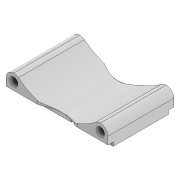
# Autodesk Inventor part: oxybeamBottom
Saved by Autodesk Inventor 2020 (Build 240168000, 168)
## iProperties
Created: 2020-05-15
Part Number: oxybeamBottom
Material: Generic
Document SubType Name: Modeling
Designer: rayan
Density: 1 g/cm^3
Appearance: Default
Author: rayan
Autodesk Inventor part; units mm, degrees
ref_plane "XZ Plane" through (0, 0, 0) normal (0, 1, 0) x (-1, 0, 0)
ref_plane "XY Plane" through (0, 0, 0) normal (0, 0, 1) x (1, 0, 0)
sketch "Sketch1" plane through (0, 0, 0) normal (0, 0, 1) x (1, 0, 0)
  circle A0 centre (0, 0) radius 1.7
  circle A1 centre (0, 0) radius 3
  dimension "d0" = 3.4
  dimension "d1" = 6
  constraints: 2 centre point, 2 coincident
  measures "d0" diameter of A0
  measures "d1" diameter of A1
extrude "Extrusion1" add sketch "Sketch1" along normal mid plane 26
sketch "Sketch2" plane through (0, 0, 13) normal (0, 0, 1) x (1, 0, 0)
  line L0 (0, 0) -> (-3, 0)
  line L1 (-3, 0) -> (-3, -8)
  line L2 (-3, -8) -> (0, -8)
  line L3 (0, -8) -> (0, 0) construction
  line L4 (0, 0) -> (3, 0)
  line L5 (3, 0) -> (3, -5)
  line L6 (3, -5) -> (0, -5)
  line L7 (0, -5) -> (0, 0) construction
  line L8 (0, -5) -> (0, -8)
  circle A0 centre (0, 0) radius 1.7 projected
  point P0 (1.7, 0)
  point P1 (-1.7, 0)
  dimension "d4" = 3
  dimension "d5" = 8
  dimension "d6" = 3
  dimension "d7" = 5
  constraints: 18 end point, 4 parallel, 3 perpendicular, 2 horizontal
  measures "d4" distance of L2.end L1.end
  measures "d5" distance of L1.end L0.end
  measures "d6" distance of L5.end L6.end
  measures "d7" distance of L4.end L5.end
extrude "Extrusion2" add sketch "Sketch2" against normal up to surface (26 mm away) contours A0 L4 L5 L6 L8 L2 L1 L0
sketch "Sketch3" plane through (0, 0, 13) normal (0, 0, 1) x (1, 0, 0)
  line L0 (-3, 0) -> (-3, -8) projected
  line L1 (3, -5) -> (3, 0) projected
  line L2 (-3, -8) -> (3, -8)
  line L3 (3, -8) -> (3, -3)
  line L4 (3, -3) -> (-3, -3)
  line L5 (-3, -3) -> (-3, -8)
  point P0 (0, 0)
  point P1 (-3, -3)
  dimension "d10" = 5
  constraints: 8 end point, 2 parallel, 1 horizontal, 1 perpendicular, 1 point on line
  measures "d10" distance of L3.end L2.end
extrude "Extrusion3" cut sketch "Sketch3" against normal blind 2.05
mirror "Mirror1" about plane through (0, 0, 0) normal (0, 0, 1) of "Extrusion3"
sketch "Sketch4" plane through (0, -8, 10.95) normal (1, 0, 0) x (0, 0, -1)
  line L0 (0, 3) -> (0, 0) projected
  line L1 (0, 0) -> (21.9, 0) projected
  line L2 (0, 0) -> (21.9, 0)
  line L3 (21.9, 0) -> (21.9, 3.5)
  line L4 (21.9, 3.5) -> (0, 3.5)
  line L5 (0, 3.5) -> (0, 0)
  line L6 (0, 3) -> (21.9, 3) construction
  line L7 (21.9, 5) -> (23.95, 5) projected
  point P0 (10.95, 8)
  point P1 (0, 1.5)
  dimension "d16" = 1.5
  constraints: 8 end point, 2 parallel, 1 horizontal, 1 perpendicular
  measures "d16" distance between parallel lines of L7 L4
extrude "Extrusion4" cut sketch "Sketch4" against normal through all both and the other way through all
sketch "Sketch5" plane through (3, 0, 13) normal (1, 0, 0) x (0, 0, -1)
  line L0 (23.95, -4.5) -> (2.05, -4.5) projected
  line L1 (2.05, -4.5) -> (5.05, -4.5)
  line L2 (23.95, -4.5) -> (23.95, -3) projected
  line L3 (23.95, -4.5) -> (20.95, -4.5)
  line L4 (2.05, -3) -> (0, -3) projected
  line L5 (26, -3) -> (23.95, -3) projected
  line L6 (2.05, -3) -> (23.95, -3)
  arc A0 (20.95, -4.5) -> (5.05, -4.5) centre (13, -24.8175) ccw
  point P0 (13, 0)
  dimension "d17" = 3
  dimension "d18" = 3
  constraints: 6 end point, 2 point on circle, 2 point on line, 1 centre point, 1 collinear, 1 tangent
  measures "d17" distance of L0.end L1.end
  measures "d18" distance of L0.start L3.end
extrude "Extrusion5" [suppressed]
fillet "Fillet1" [suppressed]
ref_plane "Work Plane1" through (17.1, 0, 0) normal (1, 0, 0) x (0, 1, 0)
mirror "Mirror2" about plane through (17.1, 0, 0) normal (1, 0, 0) of "Extrusion1", "Extrusion2", "Extrusion3", "Mirror1", "Extrusion4"
sketch "Sketch7" plane through (3, 0, 13) normal (1, 0, 0) x (0, 0, -1)
  line L0 (23.95, -4.5) -> (23.95, -3) projected
  line L1 (23.95, -3) -> (26, -3) projected
  line L2 (26, 0) -> (26, -3) projected
  line L3 (26, 0) -> (0, 0) projected
  line L4 (0, -3) -> (0, 0) projected
  line L5 (0, -3) -> (2.05, -3) projected
  line L6 (2.05, -3) -> (2.05, -4.5) projected
  line L7 (0, 3) -> (0, 0) projected
  line L8 (26, 0) -> (0, 0) projected
  line L9 (0, 0) -> (26, 0)
  line L10 (26, 0) -> (26, -1.5)
  line L11 (26, -1.5) -> (0, -1.5)
  line L12 (0, -1.5) -> (0, 0)
  line L13 (2.05, -4.5) -> (23.95, -4.5) projected
  point P0 (13, 0)
  point P1 (0, -1.5)
  dimension "d25" = 1.5
  constraints: 8 end point, 3 equal length, 1 perpendicular
  measures "d25" distance between parallel lines of L11 L5
extrude "Extrusion7" add sketch "Sketch7" along normal up to surface (28.2 mm away) contours L13 L6 L5 L4 L11 L2 L1 L0
sketch "Sketch8" plane through (3, -1.5, 13) normal (0, 1, 0) x (1, 0, 0)
  line L0 (28.2, 26) -> (28.2, 0) construction
  line L1 (0, 26) -> (28.2, 26) construction
  line L2 (0, 0) -> (0, 26) construction
  line L3 (0, 0) -> (28.2, 0) construction
  line L4 (-6, 0) -> (0, 0) construction
  line L5 (28.2, 26) -> (0, 0) construction
  line L6 (28.2, 26) -> (28.2, 0) projected
  line L7 (0, 7.2315) -> (28.2, 7.2315)
  line L8 (28.2, 7.2315) -> (28.2, 18.7685)
  line L9 (28.2, 18.7685) -> (0, 18.7685)
  line L10 (0, 18.7685) -> (0, 7.2315)
  line L11 (0, 7.2315) -> (28.2, 18.7685) construction
  line L12 (28.2, 7.2315) -> (0, 18.7685) construction
  point P0 (-3, 13)
  point P1 (14.1, 13)
  dimension "d28" = 11.537
  constraints: 14 end point, 3 midpoint, 2 parallel, 1 horizontal, 1 perpendicular, 1 point on line
  measures "d28" distance of L8.end L7.end
extrude "Extrusion8" [suppressed]
fillet "Fillet2" radius 1.5 2 edges at (31.2, -1.5, 0) (3, -1.5, 0)
fillet "Fillet3" [suppressed]
sketch "Sketch9" plane through (0, 0, -13) normal (0, 0, -1) x (-1, 0, 0)
  arc A0 (3, 0) -> (-3, 0) centre (0, 0) ccw construction
  line L0 (0, 0) -> (0, 3)
  line L1 (0, 3) -> (-1.1, 3)
  line L2 (-1.1, 3) -> (-1.1, 0) construction
  line L3 (-1.1, 0) -> (0, 0)
  circle A1 centre (-34.2, 0) radius 1.7 projected
  arc A2 (-31.2, 0) -> (-37.2, 0) centre (-34.2, 0) ccw construction
  line L4 (-34.2, 0) -> (-34.2, 3)
  line L5 (-34.2, 3) -> (-33.1, 3)
  line L6 (-33.1, 3) -> (-33.1, 0) construction
  line L7 (-33.1, 0) -> (-34.2, 0) construction
  circle A3 centre (0, 0) radius 1.7 projected
  circle A4 centre (-34.2, 0) radius 1.7 projected
  line L8 (-37.2, -3) -> (3, -3) construction
  line L9 (3, -3) -> (3, 0) projected
  arc A5 (3, 0) -> (-3, 0) centre (0, 0) ccw construction
  arc A6 (-4.5, -1.5) -> (-3, 0) centre (-4.5, 0) ccw construction
  line L10 (-4.5, -1.5) -> (-29.7, -1.5) construction
  arc A7 (-31.2, 0) -> (-29.7, -1.5) centre (-29.7, 0) ccw projected
  arc A8 (-31.2, 0) -> (-37.2, 0) centre (-34.2, 0) ccw construction
  line L11 (-37.2, -3) -> (-37.2, 0) construction
  line L12 (-34.2, 0) -> (0, 0) construction
  line L13 (0, 0) -> (0, -3)
  line L14 (0, -3) -> (-34.2, -3)
  line L15 (-34.2, -3) -> (-34.2, 0)
  arc A9 (-33.1, 3) -> (-1.1, 3) centre (-17.1, 21.3333) ccw
  line L16 (-33.1, 3) -> (-34.2, 3)
  line L17 (-1.1, 3) -> (0, 3)
  line L18 (-4.5, -1.5) -> (-29.7, -1.5) projected
  line L19 (-25.5113, -1.5) -> (-8.6887, -1.5)
  point P0 (-17.1, -3)
  point P1 (-34.2, 1.7)
  point P2 (-34.2, -1.7)
  point P3 (0, -1.7)
  point P4 (0, 1.7)
  dimension "d33" = 1.1
  dimension "d34" = 1.1
  dimension "d35" = 3
  constraints: 30 end point, 8 equal length, 6 point on circle, 3 perpendicular, 3 tangent, 2 point on line, 2 vertical, 1 centre point, 1 horizontal
  measures "d33" distance of L1.end L0.end
  measures "d34" distance of L4.end L5.end
  measures "d35" distance of L12.end L13.end
extrude "Extrusion9" add sketch "Sketch9" against normal up to surface (26 mm away) contours A3 L13 L14 A9 L1 L0 | L14 L15 A1 L4 L5 A9
extrude "Extrusion10" cut sketch "Sketch9" against normal through all contours A9 L18
fillet "Fillet4" radius 3 2 edges at (1.1, 3, 0) (33.1, 3, 0)
sketch "Sketch10" plane through (-3, -3, -13) normal (0, -1, 0) x (1, 0, 0)
  line L0 (20.1, 23.95) -> (20.1, 26) projected
  line L1 (0, 26) -> (20.1, 26) projected
  line L2 (0, 23.95) -> (0, 26) projected
  line L3 (20.1, 23.95) -> (0, 23.95) projected
  line L4 (40.2, 23.95) -> (20.1, 23.95) projected
  line L5 (40.2, 26) -> (40.2, 23.95) projected
  line L6 (20.1, 26) -> (40.2, 26) projected
  line L7 (37.2, 26) -> (37.2, 0) projected
  line L8 (37.2, 23.95) -> (27.2, 23.95)
  line L9 (37.2, 23.95) -> (47.2, 23.95) construction
  line L10 (27.2, 23.95) -> (23.7, 23.95)
  line L11 (23.7, 23.95) -> (23.7, 14.95)
  line L12 (23.7, 14.95) -> (27.2, 14.95)
  line L13 (27.2, 14.95) -> (27.2, 23.95)
  line L14 (27.2, 14.95) -> (27.2, 23.95)
  line L15 (27.2, 23.95) -> (30.7, 23.95)
  line L16 (30.7, 23.95) -> (30.7, 14.95)
  line L17 (30.7, 14.95) -> (27.2, 14.95)
  line L18 (20.1, 0) -> (20.1, 2.05) projected
  line L19 (0, 2.05) -> (20.1, 2.05) projected
  line L20 (0, 0) -> (0, 2.05) projected
  line L21 (20.1, 0) -> (0, 0) projected
  line L22 (40.2, 0) -> (20.1, 0) projected
  line L23 (40.2, 2.05) -> (40.2, 0) projected
  line L24 (20.1, 2.05) -> (40.2, 2.05) projected
  line L25 (3, 26) -> (3, 0) projected
  line L26 (3, 2.05) -> (11, 2.05)
  line L27 (3, 2.05) -> (11, 2.05) construction
  line L28 (11, 2.05) -> (7.5, 2.05)
  line L29 (7.5, 2.05) -> (7.5, 11.05)
  line L30 (7.5, 11.05) -> (11, 11.05)
  line L31 (11, 11.05) -> (11, 2.05)
  line L32 (11, 11.05) -> (11, 2.05)
  line L33 (11, 2.05) -> (14.5, 2.05)
  line L34 (14.5, 2.05) -> (14.5, 11.05)
  line L35 (14.5, 11.05) -> (11, 11.05)
  dimension "d56" = 10
  dimension "d57" = 180
  dimension "d58" = 3.5
  dimension "d59" = 9
  dimension "d60" = 3.5
  dimension "d61" = 8
  dimension "d62" = 0
  dimension "d63" = 3.5
  dimension "d64" = 9
  dimension "d65" = 3.5
  constraints: 40 end point, 8 parallel, 6 collinear, 4 horizontal, 4 perpendicular, 4 point on line
  measures "d56" distance of L8.start L8.end
  measures "d57" angle of L8 L9
  measures "d58" distance of L12.end L11.end
  measures "d59" distance of L11.end L10.end
  measures "d60" distance of L16.end L12.end
  measures "d61" distance of L26.start L26.end
  measures "d62" distance between parallel lines of L26 L27
  measures "d63" distance of L29.end L30.end
  measures "d64" distance of L28.end L29.end
  measures "d65" distance of L34.end L30.end
extrude "Extrusion11" cut sketch "Sketch10" along normal blind 10 contours L4 L13 L12 L11 | L4 L16 L17 L13 | L29 L30 L31 L19 | L31 L35 L34 L19
sketch "Sketch11" plane through (-3, -3, -13) normal (0, -1, 0) x (1, 0, 0)
  line L0 (20.1, 0) -> (20.1, 2.05) construction
  line L1 (40.2, 0) -> (20.1, 0) projected
  line L2 (40.2, 2.05) -> (40.2, 0) projected
  line L3 (20.1, 2.05) -> (40.2, 2.05) construction
  line L4 (0, 2.05) -> (7.5, 2.05) projected
  line L5 (0, 0) -> (0, 2.05) projected
  line L6 (20.1, 0) -> (0, 0) projected
  line L7 (20.1, 23.95) -> (20.1, 26) construction
  line L8 (0, 26) -> (20.1, 26) projected
  line L9 (0, 23.95) -> (0, 26) projected
  line L10 (20.1, 23.95) -> (0, 23.95) construction
  line L11 (40.2, 23.95) -> (30.7, 23.95) construction
  line L12 (40.2, 26) -> (40.2, 23.95) projected
  line L13 (20.1, 26) -> (40.2, 26) projected
  line L14 (35.5, 0) -> (38.9, 0) projected
  line L15 (4.7, 0) -> (1.3, 0) projected
  line L16 (37.188, 0) -> (37.2, 0) projected
  line L17 (37.2, 0) -> (27.2, 0)
  line L18 (35.3125, 0) -> (20.1, 0) projected
  line L19 (0, 0) -> (3, 0) projected
  line L20 (3, 0) -> (13, 0)
  line L21 (20.1, 0) -> (0, 0) projected
  line L22 (3, 0) -> (13, 0) construction
  line L23 (27.2, 0) -> (13, 0)
  line L24 (13, 0) -> (13, 26) construction
  line L25 (13, 26) -> (27.2, 26)
  line L26 (27.2, 26) -> (27.2, 0) construction
  arc A0 (27.2, 0) -> (13, 0) centre (20.1, -11.2701) ccw
  arc A1 (13, 26) -> (27.2, 26) centre (20.1, 37.2701) ccw
  line L27 (13, 26) -> (27.2, 0) construction
  line L28 (20.1, 13) -> (27.2, 13) construction
  ellipse E0 centre (20.1, 13) end of major axis (27.2, 13) minor radius 5
  line L29 (23.7, 23.95) -> (20.1, 23.95) projected
  line L30 (23.7, 23.95) -> (23.7, 14.95) projected
  line L31 (23.7, 14.95) -> (30.7, 14.95) projected
  line L32 (30.7, 14.95) -> (30.7, 23.95) projected
  line L33 (14.5, 2.05) -> (20.1, 2.05) projected
  line L34 (14.5, 2.05) -> (14.5, 11.05) projected
  line L35 (14.5, 11.05) -> (7.5, 11.05) projected
  line L36 (7.5, 11.05) -> (7.5, 2.05) projected
  point P0 (3, 13)
  point P1 (27.2, 26)
  dimension "d51" = 5
  dimension "d47" = 10
  dimension "d48" = 10
  dimension "d49" = 0
  dimension "d50" = 26
  constraints: 18 end point, 5 point on circle, 3 collinear, 2 centre point, 2 horizontal, 2 midpoint, 2 parallel, 1 coincident, 1 horizontal alignment, 1 perpendicular, 1 point on line, 1 tangent, 2 other
  measures "d47" distance of L16.end L17.end
  measures "d48" distance of L19.end L20.end
  measures "d49" distance between parallel lines of L20 L22
  measures "d50" distance of L22.end L24.end
extrude "Extrusion12" cut sketch "Sketch11" against normal through all both and the other way through all contours L1 L6 A0 | L8 L13 A1
fillet "Fillet5" radius 3 4 edges at (24.2, -2.4706, -13) (10, -2.4706, -13) (10, -2.4706, 13) (24.2, -2.4706, 13)
full round fillet "Fillet7" first side at (4.5, -3.5, -4.95) centre faces at (6.8333, -4, -1.95) second side at (11.5, -3.5, -7.95)
full round fillet "Fillet8" first side at (27.7, -4, 7.95) centre faces at (23.0333, -3.5, 1.95) second side at (20.7, -3.5, 7.95)
equation "\"d34\" = d33"
equation "\"d60\" = d58"
equation "\"d63\" = d58"
equation "\"d64\" = d59"
equation "\"d65\" = d58"
body "Solid1"
